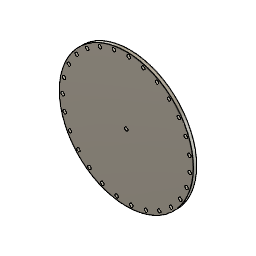
盘新 (Autodesk Fusion 360 design; units mm, degrees)
part number: 2025-10-23-15-16-33-441
Autodesk Fusion 360 part; units mm, degrees
sketch "草图1" plane through (0, 0, 0) normal (0, 0, 1) x (1, 0, 0)
  circle A0 centre (0, 0) radius 60
  circle A1 centre (-35, 45) radius 1.5
  circle A2 centre (-44.4343, 35.7155) radius 1.5
  circle A3 centre (-51.4731, 24.5055) radius 1.5
  circle A4 centre (-55.737, 11.9744) radius 1.5
  circle A5 centre (-56.9961, -1.2022) radius 1.5
  circle A6 centre (-55.1825, -14.314) radius 1.5
  circle A7 centre (-50.394, -26.6541) radius 1.5
  circle A8 centre (-42.8888, -37.5573) radius 1.5
  circle A9 centre (-33.0714, -46.4358) radius 1.5
  circle A10 centre (-21.4711, -52.8109) radius 1.5
  circle A11 centre (-8.7134, -56.339) radius 1.5
  circle A12 centre (4.5142, -56.8298) radius 1.5
  circle A13 centre (17.4983, -54.2569) radius 1.5
  circle A14 centre (29.5392, -48.759) radius 1.5
  circle A15 centre (39.9875, -40.6325) radius 1.5
  circle A16 centre (48.2801, -30.3155) radius 1.5
  circle A17 centre (53.97, -18.3641) radius 1.5
  circle A18 centre (56.7503, -5.4228) radius 1.5
  circle A19 centre (56.4711, 7.8109) radius 1.5
  circle A20 centre (53.1476, 20.6235) radius 1.5
  circle A21 centre (46.9589, 32.3243) radius 1.5
  circle A22 centre (38.2387, 42.2824) radius 1.5
  circle A23 centre (27.4569, 49.9612) radius 1.5
  circle A24 centre (15.195, 54.9464) radius 1.5
  circle A25 centre (2.1139, 56.9696) radius 1.5
  circle A26 centre (-11.0812, 55.9214) radius 1.5
  circle A27 centre (-23.6789, 51.8586) radius 1.5
  circle A28 centre (0, 0) radius 1.5
  dimension "d1" = 120
  dimension "d2" = 3
  dimension "d4" = 360
  dimension "d5" = 3
  constraint coincident A0.centre A28.centre
  measures "d1" diameter of A0
  measures "d2" diameter of A1
  measures "d5" diameter of A28
extrude "拉伸1" add sketch "草图1" along normal blind 3
